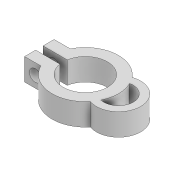
# Autodesk Inventor part: Spring_hook
Saved by Autodesk Inventor 2022 (Build 260153000, 153)
## iProperties
Created: 2022-07-09
Part Number: Spring_hook
Material: Generic
Document SubType Name: Modeling
Designer: dell
Density: 1 g/cm^3
Appearance: Default
Author: dell
Autodesk Inventor part; units mm, degrees
ref_plane "YZ Plane" through (0, 0, 0) normal (1, 0, 0) x (0, 1, 0)
ref_plane "XZ Plane" through (0, 0, 0) normal (0, 1, 0) x (-1, 0, 0)
ref_plane "XY Plane" through (0, 0, 0) normal (0, 0, 1) x (1, 0, 0)
sketch "Sketch1" plane through (0, 0, 0) normal (0, 1, 0) x (-1, 0, 0)
  circle A0 centre (0, 0) radius 6
  circle A1 centre (0, 0) radius 9
  line L0 (4.4721, 4) -> (12.4721, 4)
  line L1 (12.4721, 4) -> (12.4721, 1)
  line L2 (12.4721, 1) -> (4.4721, 1)
  line L3 (4.4721, 1) -> (4.4721, 4)
  line L4 (4.4721, -4) -> (12.4721, -4)
  line L5 (12.4721, -4) -> (12.4721, -1)
  line L6 (12.4721, -1) -> (4.4721, -1)
  line L7 (4.4721, -1) -> (4.4721, -4)
  circle A2 centre (-9, 0) radius 4
  circle A3 centre (-9, 0) radius 6
  point P0 (-8.1111, -3.9)
  point P1 (-8.1111, 3.9)
  point P2 (5.9161, 1)
  point P3 (8.0623, 4)
  point P4 (-7, 5.6569)
  point P5 (-7, -5.6569)
  point P6 (8.0623, -4)
  point P7 (5.9161, -1)
  dimension "d0" = 12
  dimension "d1" = 3
  dimension "d2" = 3
  dimension "d3" = 3
  dimension "d4" = 1
  dimension "d5" = 1
  dimension "d6" = 8
  dimension "d7" = 8
  dimension "d8" = 8
  dimension "d9" = 2
  constraints: 16 end point, 4 parallel, 3 centre point, 2 horizontal, 2 perpendicular, 2 point on circle, 1 coincident, 3 other
  measures "d0" diameter of A0
  measures "d2" distance between parallel lines of L0 L2
  measures "d3" distance between parallel lines of L4 L6
  measures "d4" distance from line of point (0, 0) L2
  measures "d5" distance from line of point (0, 0) L6
  measures "d6" distance between parallel lines of L3 L1
  measures "d7" distance between parallel lines of L7 L5
  measures "d8" diameter of A2
  measures "d9" radial gap between concentric circles of A2 A3
extrude "Extrusion1" add sketch "Sketch1" along normal blind 6 contours A0 L0 A1 L2 | L6 A1 L4 A0 | A0 A3 A1 L0 | A1 L0 L1 L2 | L4 A1 A3 A0 | L6 L5 L4 A1 | A0 A2 A1 A3 | A3 A1 A2 A0 | A0 A2 A1 | A1 A2 A3
sketch "Sketch2" plane through (-12.4721, 0, 4) normal (0, 0, 1) x (1, 0, 0)
  line L0 (0, 0) -> (4.4099, 0) projected
  line L1 (4.4099, 0) -> (4.4099, 6) projected
  line L2 (0, 6) -> (4.4099, 6) projected
  line L3 (0, 0) -> (0, 6) projected
  circle A0 centre (2.8989, 3) radius 1.6
  point P0 (12.4721, 0)
  dimension "d12" = 3.2
  constraints: 1 centre point
  measures "d12" diameter of A0
extrude "Extrusion2" cut sketch "Sketch2" against normal blind 10 contours A0 L1 | L1 A0
body "Solid1"
